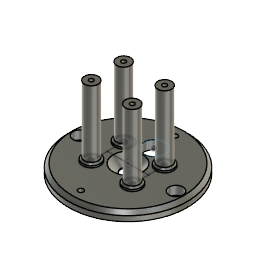
WeatherLox-Air-Adapter (Autodesk Fusion 360 design; units mm, degrees)
Autodesk Fusion 360 part; units mm, degrees
sketch "Skizze1" plane through (0, 0, 0) normal (0, 0, 1) x (1, 0, 0)
  circle A0 centre (0, 0) radius 34
  line L0 (0, 0) -> (0, 27)
  line L1 (0, 0) -> (0, -27)
  line L2 (34, 0) -> (27.5, 0)
  line L3 (27.5, 0) -> (25.5, 0)
  circle A1 centre (27.5, 0) radius 4
  line L4 (-34, 0) -> (-27.5, 0)
  circle A2 centre (-27.5, 0) radius 4
  dimension "d1" = 68
  dimension "d9" = 27
  dimension "d10" = 27
  dimension "d81" = 8
  dimension "d83" = 8
  constraint coincident A0.centre L0.start
  constraint coincident A0 L2.start
  constraint horizontal L2
  constraint coincident L2.end L3.start
  constraint coincident A0 L4.start
  constraint horizontal L4
  constraint coincident L4.end A2.centre
  measures "d1" diameter of A0
  measures "d9" distance of A0.centre L0.end
  measures "d10" distance of A0.centre L1.end
  measures "d81" diameter of A1
  measures "d83" diameter of A2
extrude "Extrusion1" add sketch "Skizze1" along normal blind 5 contours A0 | A1 | A2
sketch "Skizze2" plane through (0, 0, 5) normal (0, 0, 1) x (-1, 0, 0)
  circle A0 centre (0, 0) radius 34
  line L0 (0, 0) -> (11.75, 0)
  line L1 (11.75, 0) -> (11.75, -9.25)
  line L2 (11.75, 0) -> (11.75, 9.25)
  line L3 (0, 0) -> (-11.75, 0)
  line L4 (-11.75, 0) -> (-11.75, 9.25)
  line L5 (-11.75, 0) -> (-11.75, -9.25)
  circle A1 centre (-11.75, 9.25) radius 4
  circle A2 centre (-11.75, -9.25) radius 4
  circle A3 centre (11.75, 9.25) radius 4
  circle A4 centre (11.75, -9.25) radius 4
  circle A5 centre (0, -15) radius 6
  circle A6 centre (11.75, 9.25) radius 5
  circle A7 centre (11.75, -9.25) radius 5
  circle A8 centre (-11.75, -9.25) radius 5
  circle A9 centre (-11.75, 9.25) radius 5
  point P0 (0, -15)
  dimension "d39" = 11.75
  dimension "d40" = 9.25
  dimension "d41" = 9.25
  dimension "d42" = 11.75
  dimension "d43" = 9.25
  dimension "d44" = 9.25
  dimension "d45" = 8
  dimension "d46" = 8
  dimension "d47" = 8
  dimension "d48" = 8
  dimension "d79" = 12
  dimension "d90" = 10
  dimension "d91" = 10
  dimension "d92" = 10
  dimension "d93" = 10
  constraint coincident A0.centre L0.start
  constraint horizontal L0
  constraint perpendicular L0 L1
  constraint perpendicular L0 L2
  constraint parallel L0 L3
  constraint perpendicular L3 L4
  constraint perpendicular L3 L5
  constraint coincident L4.end A1.centre
  constraint coincident L5.end A2.centre
  constraint coincident L2.end A3.centre
  constraint coincident L1.end A4.centre
  constraint coincident P0 A5.centre
  constraint concentric A3 A6
  constraint concentric A4 A7
  constraint concentric A2 A8
  constraint concentric A1 A9
  measures "d39" distance of A0.centre L0.end
  measures "d40" distance of L0.end L1.end
  measures "d41" distance of L0.end L2.end
  measures "d42" distance of A0.centre L3.end
  measures "d43" distance of L3.end L4.end
  measures "d44" distance of L3.end L5.end
  measures "d45" diameter of A1
  measures "d46" diameter of A2
  measures "d47" diameter of A3
  measures "d48" diameter of A4
  measures "d79" diameter of A5
  measures "d90" diameter of A6
  measures "d91" diameter of A7
  measures "d92" diameter of A8
  measures "d93" diameter of A9
hole "Bohrung1" at (0, 0, 5) direction (0, 0, -1) diameter 8 depth 15 tip angle 118 countersink diameter 17 countersink angle 90
extrude "Extrusion7" add sketch "Skizze2" along normal blind 40 contours A1 | A2 | A3 | A4
hole "Bohrung2" at (0, -27, 0) direction (0, 0, 1) diameter 3 depth 15 tip angle 118 countersink diameter 6 countersink angle 90
hole "Bohrung3" at (0, 27, 0) direction (0, 0, 1) diameter 3 depth 15 tip angle 118 countersink diameter 6 countersink angle 90
sketch "Skizze4" plane through (0, 0, 45) normal (0, 0, 1) x (-1, 0, 0)
  circle A0 centre (11.75, -9.25) radius 4
  point P0 (11.75, -9.25)
  point P1 (-11.749, -9.25)
  point P2 (11.75, 9.2641)
  point P3 (-11.749, 9.2641)
  constraint coincident P0 A0.centre
hole "Bohrung4" at (-11.75, 9.25, 45) direction (0, 0, -1) diameter 2.5 depth 4 tip angle 118
hole "Bohrung5" at (-11.75, -9.2641, 45) direction (0, 0, -1) diameter 2.5 depth 4 tip angle 118
hole "Bohrung6" at (11.749, -9.2641, 45) direction (0, 0, -1) diameter 2.5 depth 4 tip angle 118
hole "Bohrung7" at (11.749, 9.25, 45) direction (0, 0, -1) diameter 2.5 depth 4 tip angle 118
extrude "Extrusion8" cut sketch "Skizze1" along normal blind 7 contours A1
extrude "Extrusion9" cut sketch "Skizze1" along normal blind 7 contours A2
extrude "Extrusion10" cut sketch "Skizze2" against normal blind 5 contours A5
extrude "Extrusion11" add sketch "Skizze2" along normal blind 2 contours A9
chamfer "Fase1" distance 1 angle 45 1 edges at (16.4116, -7.4419, 7)
extrude "Extrusion12" add sketch "Skizze2" along normal blind 2 contours A6
chamfer "Fase2" distance 1 angle 45 1 edges at (-7.0884, -7.4419, 7)
extrude "Extrusion13" add sketch "Skizze2" along normal blind 2 contours A7
extrude "Extrusion14" add sketch "Skizze2" along normal blind 2 contours A8
chamfer "Fase3" distance 1 angle 45 1 edges at (-7.0884, 11.0581, 7)
chamfer "Fase4" distance 1 angle 45 1 edges at (16.4116, 11.0581, 7)
sketch "Skizze5" plane through (0, 0, 5) normal (0, 0, 1) x (-1, 0, 0)
  line L0 (-5.2362, -23.9768) -> (5.156, -24.023)
  line L1 (5.156, -24.023) -> (10.3922, -15.0463)
  line L2 (10.3922, -15.0463) -> (5.2362, -6.0232)
  line L3 (5.2362, -6.0232) -> (-5.156, -5.977)
  line L4 (-5.156, -5.977) -> (-10.3922, -14.9537)
  line L5 (-10.3922, -14.9537) -> (-5.2362, -23.9768)
  point P0 (0, -15)
  dimension "d106" = 9
  measures "d106" distance of P0 L5
extrude "Extrusion15" cut sketch "Skizze5" along normal blind 5
chamfer "Fase5" distance 2 angle 45 1 edges at (-31.6991, -12.2949, 5)
sketch "Skizze6" plane through (0, 0, 0) normal (0, 1, 0) x (1, 0, 0)
sketch "Skizze7" plane through (0, 0, 0) normal (1, 0, 0) x (0, 1, 0)
extrude "Extrusion2" [suppressed]
extrude "Extrusion3" [suppressed]
extrude "Extrusion4" [suppressed]
extrude "Extrusion5" [suppressed]
extrude "Extrusion6" [suppressed]
